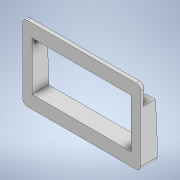
# Autodesk Inventor part: electricalCoverGasket02
Saved by Autodesk Inventor 2021.1 (Build 251245000, 245)
## iProperties
Created: 2020-08-29
Part Number: electricalCoverGasket02
Material: Generic
Document SubType Name: Modeling
Designer: robst
Density: 1 g/cm^3
Appearance: Default
Author: robst
Autodesk Inventor part; units mm, degrees
ref_plane "YZ Plane" through (0, 0, 0) normal (1, 0, 0) x (0, 1, 0)
ref_plane "XZ Plane" through (0, 0, 0) normal (0, 1, 0) x (-1, 0, 0)
sketch "Sketch1" plane through (0, 0, 0) normal (1, 0, 0) x (0, 1, 0)
  line L0 (0, 0) -> (0, 12.7)
  line L1 (0, 0) -> (-101.6, 0) construction
  arc A0 (-101.6, 0) -> (0, 0) centre (-50.8, 607.4796) ccw
  line L2 (-50.8, -2.1204) -> (-50.8, 0) construction
  line L3 (0, 12.7) -> (101.6, 12.7) construction
  arc A1 (0, 12.7) -> (101.6, 12.7) centre (50.8, 620.1796) ccw
  line L4 (19.685, 15.1842) -> (-57.785, 15.1842)
  line L5 (-57.785, 15.1842) -> (-57.785, -2.0803)
  line L6 (19.685, 15.1842) -> (19.685, 11.3742)
  dimension "d5" = 609.6
  dimension "d6" = 101.6
  dimension "d7" = 609.6
  dimension "d24" = 12.7
  dimension "d26" = 77.47
  dimension "d28" = 57.785
  dimension "d29" = 3.81
  constraints: 14 end point, 7 point on circle, 3 horizontal, 2 centre point, 2 perpendicular, 1 midpoint, 1 vertical
  measures "d5" radius of A0
  measures "d6" distance of L0.end L3.end
  measures "d7" radius of A1
  measures "d24" distance of L0.start L0.end
  measures "d26" distance of L4.start L4.end
  measures "d28" distance between parallel lines of L0 L5
  measures "d29" distance of L4.start L6.end
extrude "Extrusion3" add sketch "Sketch1" along normal mid plane 122.428
sketch "Sketch5" plane through (0, 0, 0) normal (0, 0, 1) x (1, 0, 0)
  line L0 (-61.214, 19.685) -> (61.214, 19.685) projected
  line L1 (-61.214, 0) -> (61.214, 0) projected
  line L2 (61.214, 0) -> (61.214, 19.685)
  line L3 (-61.214, 19.685) -> (-61.214, 0)
  line L4 (61.214, 12.065) -> (-61.214, 12.065) construction
  line L5 (-61.214, -57.785) -> (-61.214, 19.685) construction
  line L6 (21.5694, 8.255) -> (21.5694, 14.9734)
  line L7 (21.5694, 14.9734) -> (24.1259, 14.9734)
  line L8 (24.1259, 14.9734) -> (24.1259, 15.875)
  line L9 (24.1259, 15.875) -> (18.0002, 15.875)
  line L10 (18.0002, 15.875) -> (18.0002, 14.9734)
  line L11 (18.0002, 14.9734) -> (20.5567, 14.9734)
  line L12 (20.5567, 14.9734) -> (20.5567, 8.255)
  line L13 (20.5567, 8.255) -> (21.5694, 8.255)
  spline S0 degree 2 poles (11.8314, 15.0043) (11.3991, 14.498) (10.9175, 13.016) (10.9175, 12.065) knots 0 0 0 1 2 2 2
  spline S1 degree 2 poles (10.9175, 12.065) (10.9175, 11.1387) (11.3868, 9.6382) (11.8314, 9.1319) knots 0 0 0 1 2 2 2
  spline S2 degree 2 poles (11.8314, 9.1319) (12.3007, 8.6008) (13.5419, 8.0944) (14.289, 8.0944) knots 0 0 0 1 2 2 2
  spline S3 degree 2 poles (14.289, 8.0944) (15.0609, 8.0944) (16.2959, 8.6193) (16.7467, 9.1319) knots 0 0 0 1 2 2 2
  spline S4 degree 2 poles (16.7467, 9.1319) (17.1851, 9.6382) (17.6544, 11.1264) (17.6544, 12.065) knots 0 0 0 1 2 2 2
  spline S5 degree 2 poles (17.6544, 12.065) (17.6544, 13.0221) (17.179, 14.4794) (16.7405, 15.0043) knots 0 0 0 1 2 2 2
  spline S6 degree 2 poles (16.7405, 15.0043) (16.2959, 15.5107) (15.0547, 16.0356) (14.289, 16.0356) knots 0 0 0 1 2 2 2
  spline S7 degree 2 poles (14.289, 16.0356) (13.511, 16.0356) (12.2636, 15.4921) (11.8314, 15.0043) knots 0 0 0 1 2 2 2
  spline S8 degree 2 poles (11.9734, 12.065) (11.9734, 12.8184) (12.3007, 13.9854) (12.5971, 14.3683) knots 0 0 0 1 2 2 2
  spline S9 degree 2 poles (12.5971, 14.3683) (12.8997, 14.7635) (13.7518, 15.1587) (14.2829, 15.1587) knots 0 0 0 1 2 2 2
  spline S10 degree 2 poles (14.2829, 15.1587) (14.8324, 15.1587) (15.6599, 14.7758) (15.9748, 14.3683) knots 0 0 0 1 2 2 2
  spline S11 degree 2 poles (15.9748, 14.3683) (16.2774, 13.9793) (16.5985, 12.806) (16.5985, 12.065) knots 0 0 0 1 2 2 2
  spline S12 degree 2 poles (16.5985, 12.065) (16.5985, 10.5645) (15.3388, 8.9713) (14.2829, 8.9713) knots 0 0 0 1 2 2 2
  spline S13 degree 2 poles (14.2829, 8.9713) (13.2269, 8.9713) (11.9734, 10.5645) (11.9734, 12.065) knots 0 0 0 1 2 2 2
  spline S14 degree 2 poles (4.9894, 13.5779) (4.9894, 13.0839) (5.3414, 12.1947) (5.6563, 11.8859) knots 0 0 0 1 2 2 2
  spline S15 degree 2 poles (5.6563, 11.8859) (6.0515, 11.4969) (7.1198, 11.0955) (7.9349, 11.0955) knots 0 0 0 1 2 2 2
  line L14 (7.9349, 11.0955) -> (8.7933, 11.0955)
  line L15 (8.7933, 11.0955) -> (8.7933, 8.255)
  line L16 (8.7933, 8.255) -> (9.806, 8.255)
  line L17 (9.806, 8.255) -> (9.806, 15.875)
  line L18 (9.806, 15.875) -> (7.8917, 15.875)
  spline S16 degree 2 poles (7.8917, 15.875) (7.2124, 15.875) (6.2615, 15.6527) (5.8972, 15.3995) knots 0 0 0 1 2 2 2
  spline S17 degree 2 poles (5.8972, 15.3995) (5.4711, 15.1093) (4.9894, 14.2139) (4.9894, 13.5779) knots 0 0 0 1 2 2 2
  spline S18 degree 2 poles (6.0454, 13.547) (6.0454, 13.9422) (6.3171, 14.5227) (6.5949, 14.7079) knots 0 0 0 1 2 2 2
  spline S19 degree 2 poles (6.5949, 14.7079) (6.8358, 14.8685) (7.478, 14.9981) (7.9535, 14.9981) knots 0 0 0 1 2 2 2
  line L19 (7.9535, 14.9981) -> (8.7933, 14.9981)
  line L20 (8.7933, 14.9981) -> (8.7933, 11.96)
  line L21 (8.7933, 11.96) -> (8.1017, 11.96)
  spline S20 degree 2 poles (8.1017, 11.96) (7.4841, 11.96) (6.7246, 12.1576) (6.4776, 12.417) knots 0 0 0 1 2 2 2
  spline S21 degree 2 poles (6.4776, 12.417) (6.2491, 12.6455) (6.0454, 13.1827) (6.0454, 13.547) knots 0 0 0 1 2 2 2
  line L22 (1.0745, 16.2146) -> (4.057, 6.6001)
  line L23 (4.057, 6.6001) -> (4.9215, 6.6001)
  line L24 (4.9215, 6.6001) -> (1.9513, 16.2146)
  line L25 (1.9513, 16.2146) -> (1.0745, 16.2146)
  spline S22 degree 2 poles (-5.15, 10.5953) (-5.15, 10.0272) (-4.7177, 9.1566) (-4.3596, 8.8725) knots 0 0 0 1 2 2 2
  spline S23 degree 2 poles (-4.3596, 8.8725) (-3.9273, 8.5391) (-2.9455, 8.255) (-2.1674, 8.255) knots 0 0 0 1 2 2 2
  line L26 (-2.1674, 8.255) -> (0.0185, 8.255)
  line L27 (0.0185, 8.255) -> (0.0185, 15.875)
  line L28 (0.0185, 15.875) -> (-2.0007, 15.875)
  spline S24 degree 2 poles (-2.0007, 15.875) (-2.8158, 15.875) (-3.6309, 15.77) (-4.0014, 15.5662) knots 0 0 0 1 2 2 2
  spline S25 degree 2 poles (-4.0014, 15.5662) (-4.4152, 15.3501) (-4.7918, 14.64) (-4.7918, 14.1583) knots 0 0 0 1 2 2 2
  spline S26 degree 2 poles (-4.7918, 14.1583) (-4.7918, 13.6211) (-4.2237, 12.769) (-3.7235, 12.5281) knots 0 0 0 1 2 2 2
  line L29 (-3.7235, 12.5281) -> (-3.7235, 12.4911)
  spline S27 degree 2 poles (-3.7235, 12.4911) (-4.4028, 12.3058) (-5.15, 11.324) (-5.15, 10.5953) knots 0 0 0 1 2 2 2
  spline S28 degree 2 poles (-4.0941, 10.5521) (-4.0941, 10.9844) (-3.8471, 11.5401) (-3.4765, 11.7377) knots 0 0 0 1 2 2 2
  spline S29 degree 2 poles (-3.4765, 11.7377) (-3.2357, 11.8612) (-2.6676, 11.9353) (-2.1427, 11.9353) knots 0 0 0 1 2 2 2
  line L30 (-2.1427, 11.9353) -> (-0.9942, 11.9353)
  line L31 (-0.9942, 11.9353) -> (-0.9942, 9.1195)
  line L32 (-0.9942, 9.1195) -> (-1.8155, 9.1195)
  spline S30 degree 2 poles (-1.8155, 9.1195) (-2.4824, 9.1195) (-3.2481, 9.243) (-3.5445, 9.4406) knots 0 0 0 1 2 2 2
  spline S31 degree 2 poles (-3.5445, 9.4406) (-3.8285, 9.6444) (-4.0941, 10.1507) (-4.0941, 10.5521) knots 0 0 0 1 2 2 2
  spline S32 degree 2 poles (-3.7359, 14.0163) (-3.7359, 14.288) (-3.5506, 14.6956) (-3.3469, 14.8129) knots 0 0 0 1 2 2 2
  spline S33 degree 2 poles (-3.3469, 14.8129) (-3.0999, 14.9487) (-2.5009, 15.0105) (-1.9637, 15.0105) knots 0 0 0 1 2 2 2
  line L33 (-1.9637, 15.0105) -> (-0.9942, 15.0105)
  line L34 (-0.9942, 15.0105) -> (-0.9942, 12.7813)
  line L35 (-0.9942, 12.7813) -> (-2.1427, 12.7813)
  spline S34 degree 2 poles (-2.1427, 12.7813) (-2.6182, 12.7813) (-3.069, 12.8801) (-3.3098, 13.0345) knots 0 0 0 1 2 2 2
  spline S35 degree 2 poles (-3.3098, 13.0345) (-3.5445, 13.1827) (-3.7359, 13.6582) (-3.7359, 14.0163) knots 0 0 0 1 2 2 2
  line L36 (-5.3352, 8.255) -> (-7.9041, 15.875)
  line L37 (-7.9041, 15.875) -> (-9.1514, 15.875)
  line L38 (-9.1514, 15.875) -> (-11.7202, 8.255)
  line L39 (-11.7202, 8.255) -> (-10.6519, 8.255)
  line L40 (-10.6519, 8.255) -> (-9.9603, 10.3854)
  line L41 (-9.9603, 10.3854) -> (-7.0519, 10.3854)
  line L42 (-7.0519, 10.3854) -> (-6.3603, 8.255)
  line L43 (-6.3603, 8.255) -> (-5.3352, 8.255)
  line L44 (-9.6825, 11.2499) -> (-8.503, 14.8376)
  line L45 (-8.503, 14.8376) -> (-7.3298, 11.2499)
  line L46 (-7.3298, 11.2499) -> (-9.6825, 11.2499)
  spline S36 degree 2 poles (-15.5179, 8.1191) (-14.7769, 8.1191) (-13.5233, 8.6193) (-13.0664, 9.1195) knots 0 0 0 1 2 2 2
  spline S37 degree 2 poles (-13.0664, 9.1195) (-12.6094, 9.6135) (-12.1093, 11.0955) (-12.1093, 12.0588) knots 0 0 0 1 2 2 2
  spline S38 degree 2 poles (-12.1093, 12.0588) (-12.1093, 13.016) (-12.5971, 14.4362) (-13.0602, 14.9611) knots 0 0 0 1 2 2 2
  spline S39 degree 2 poles (-13.0602, 14.9611) (-13.5172, 15.4736) (-14.7645, 16.0109) (-15.5364, 16.0109) knots 0 0 0 1 2 2 2
  spline S40 degree 2 poles (-15.5364, 16.0109) (-15.9193, 16.0109) (-16.5923, 15.8997) (-16.8764, 15.8132) knots 0 0 0 1 2 2 2
  spline S41 degree 2 poles (-16.8764, 15.8132) (-17.1234, 15.733) (-17.6359, 15.5045) (-17.8891, 15.3686) knots 0 0 0 1 2 2 2
  line L47 (-17.8891, 15.3686) -> (-17.8891, 14.146)
  line L48 (-17.8891, 14.146) -> (-17.8088, 14.146)
  spline S42 degree 2 poles (-17.8088, 14.146) (-17.673, 14.2695) (-17.2531, 14.6153) (-16.9505, 14.782) knots 0 0 0 1 2 2 2
  spline S43 degree 2 poles (-16.9505, 14.782) (-16.6603, 14.9426) (-15.9748, 15.1463) (-15.5302, 15.1463) knots 0 0 0 1 2 2 2
  spline S44 degree 2 poles (-15.5302, 15.1463) (-15.0424, 15.1463) (-14.1717, 14.745) (-13.8444, 14.3621) knots 0 0 0 1 2 2 2
  spline S45 degree 2 poles (-13.8444, 14.3621) (-13.5233, 13.9731) (-13.1652, 12.7937) (-13.1652, 12.0588) knots 0 0 0 1 2 2 2
  spline S46 degree 2 poles (-13.1652, 12.0588) (-13.1652, 11.2746) (-13.5419, 10.1446) (-13.8691, 9.7555) knots 0 0 0 1 2 2 2
  spline S47 degree 2 poles (-13.8691, 9.7555) (-14.1902, 9.3789) (-15.0486, 8.996) (-15.5302, 8.996) knots 0 0 0 1 2 2 2
  spline S48 degree 2 poles (-15.5302, 8.996) (-15.9687, 8.996) (-16.7158, 9.2121) (-17.0061, 9.3727) knots 0 0 0 1 2 2 2
  spline S49 degree 2 poles (-17.0061, 9.3727) (-17.2839, 9.5332) (-17.6977, 9.8667) (-17.815, 9.984) knots 0 0 0 1 2 2 2
  line L49 (-17.815, 9.984) -> (-17.8891, 9.984)
  line L50 (-17.8891, 9.984) -> (-17.8891, 8.7737)
  spline S50 degree 2 poles (-17.8891, 8.7737) (-17.6359, 8.6564) (-17.1913, 8.4403) (-16.8764, 8.3415) knots 0 0 0 1 2 2 2
  spline S51 degree 2 poles (-16.8764, 8.3415) (-16.5429, 8.2303) (-15.9748, 8.1191) (-15.5179, 8.1191) knots 0 0 0 1 2 2 2
  line L51 (-24.3914, 8.255) -> (-23.0761, 8.255)
  line L52 (-23.0761, 8.255) -> (-20.2912, 11.7995)
  line L53 (-20.2912, 11.7995) -> (-19.8466, 11.2993)
  line L54 (-19.8466, 11.2993) -> (-19.8466, 8.255)
  line L55 (-19.8466, 8.255) -> (-18.8339, 8.255)
  line L56 (-18.8339, 8.255) -> (-18.8339, 15.875)
  line L57 (-18.8339, 15.875) -> (-19.8466, 15.875)
  line L58 (-19.8466, 15.875) -> (-19.8466, 12.3738)
  line L59 (-19.8466, 12.3738) -> (-22.9712, 15.875)
  line L60 (-22.9712, 15.875) -> (-24.2062, 15.875)
  line L61 (-24.2062, 15.875) -> (-21.0507, 12.4726)
  line L62 (-21.0507, 12.4726) -> (-24.3914, 8.255)
  point P0 (0, 0)
  dimension "d41" = 7.62
  constraints: 6 end point, 1 horizontal
  measures "d41" distance between parallel lines of L4 L0
emboss "Emboss3" sketch "Sketch5" operation cut depth 1.016 direction (0, 0, -1) wrap yes faces at (20.4047, 10.9309, 11.8848) contours L13 L12 L11 L10 L9 L8 L7 L6 | S7 S6 S5 S4 S3 S2 S1 S0 | S17 S16 L18 L17 L16 L15 L14 S15 S14 | L25 L24 L23 L22 | S27 L29 S26 S25 S24 L28 L27 L26 S23 S22 | L43 L42 L41 L40 L39 L38 L37 L36 | S51 S50 L50 L49 S49 S48 S47 S46 S45 S44 S43 S42 L48 L47 S41 S40 S39 S38 S37 S36 | L62 L61 L60 L59 L58 L57 L56 L55 L54 L53 L52 L51
ref_plane "Work Plane3" through (0, -50.8, -2.1204) normal (0, 0, 1) x (1, 0, 0)
sketch "Sketch8" plane through (-61.214, -57.785, 15.1842) normal (0, 0, 1) x (1, 0, 0)
  line L0 (122.428, 57.785) -> (0, 57.785) projected
  line L1 (61.214, 57.785) -> (61.214, 0) construction
  line L2 (0, 0) -> (122.428, 0) construction
  line L3 (9.779, 13.335) -> (112.649, 13.335)
  line L4 (112.649, 13.335) -> (112.649, 64.135)
  line L5 (112.649, 64.135) -> (9.779, 64.135)
  line L6 (9.779, 64.135) -> (9.779, 13.335)
  line L7 (9.779, 13.335) -> (112.649, 64.135) construction
  line L8 (112.649, 13.335) -> (9.779, 64.135) construction
  point P0 (61.214, 38.735)
  dimension "d36" = 50.8
  dimension "d37" = 102.87
  dimension "d38" = 13.335
  constraints: 14 end point, 3 midpoint, 2 parallel, 2 perpendicular, 1 point on line
  measures "d36" distance of L5.end L3.start
  measures "d37" distance between parallel lines of L4 L6
  measures "d38" distance between parallel lines of L2 L3
extrude "Extrusion4" cut sketch "Sketch8" against normal through all
sketch "Sketch9" plane through (0, -50.8, -2.1204) normal (0, 0, 1) x (1, 0, 0)
  line L0 (-61.214, -6.985) -> (61.214, -6.985) projected
  line L1 (-51.435, 6.35) -> (51.435, 6.35) projected
  line L2 (-51.435, 6.35) -> (-51.435, 57.15) construction
  line L3 (-51.435, 6.35) -> (-51.435, -6.985) construction
  line L4 (-61.214, -6.985) -> (61.214, -6.985) construction
  line L5 (51.435, 6.35) -> (-51.435, 6.35) construction
  line L6 (51.435, 6.35) -> (51.435, -6.985) construction
  line L7 (51.435, -0.3175) -> (-51.435, -0.3175) construction
  spline S0 degree 2 poles (7.604, -2.0321) (7.604, -2.6949) (8.1083, -3.7107) (8.5262, -4.0421) knots 0 0 0 1 2 2 2
  spline S1 degree 2 poles (8.5262, -4.0421) (9.0305, -4.4311) (10.176, -4.7625) (11.0837, -4.7625) knots 0 0 0 1 2 2 2
  line L8 (11.0837, -4.7625) -> (13.634, -4.7625)
  line L9 (13.634, -4.7625) -> (13.634, 4.1275)
  line L10 (13.634, 4.1275) -> (11.2782, 4.1275)
  spline S2 degree 2 poles (11.2782, 4.1275) (10.3272, 4.1275) (9.3763, 4.005) (8.944, 3.7673) knots 0 0 0 1 2 2 2
  spline S3 degree 2 poles (8.944, 3.7673) (8.4613, 3.5151) (8.0219, 2.6867) (8.0219, 2.1247) knots 0 0 0 1 2 2 2
  spline S4 degree 2 poles (8.0219, 2.1247) (8.0219, 1.498) (8.6847, 0.5038) (9.2682, 0.2228) knots 0 0 0 1 2 2 2
  line L11 (9.2682, 0.2228) -> (9.2682, 0.1796)
  spline S5 degree 2 poles (9.2682, 0.1796) (8.4758, -0.0365) (7.604, -1.182) (7.604, -2.0321) knots 0 0 0 1 2 2 2
  spline S6 degree 2 poles (8.836, -2.0825) (8.836, -1.5782) (9.1241, -0.9299) (9.5564, -0.6993) knots 0 0 0 1 2 2 2
  spline S7 degree 2 poles (9.5564, -0.6993) (9.8374, -0.5552) (10.5001, -0.4688) (11.1125, -0.4688) knots 0 0 0 1 2 2 2
  line L12 (11.1125, -0.4688) -> (12.4525, -0.4688)
  line L13 (12.4525, -0.4688) -> (12.4525, -3.7539)
  line L14 (12.4525, -3.7539) -> (11.4943, -3.7539)
  spline S8 degree 2 poles (11.4943, -3.7539) (10.7163, -3.7539) (9.8229, -3.6098) (9.4771, -3.3793) knots 0 0 0 1 2 2 2
  spline S9 degree 2 poles (9.4771, -3.3793) (9.1457, -3.1416) (8.836, -2.5508) (8.836, -2.0825) knots 0 0 0 1 2 2 2
  spline S10 degree 2 poles (9.2538, 1.959) (9.2538, 2.276) (9.4699, 2.7515) (9.7077, 2.8884) knots 0 0 0 1 2 2 2
  spline S11 degree 2 poles (9.7077, 2.8884) (9.9958, 3.0469) (10.6947, 3.1189) (11.3214, 3.1189) knots 0 0 0 1 2 2 2
  line L15 (11.3214, 3.1189) -> (12.4525, 3.1189)
  line L16 (12.4525, 3.1189) -> (12.4525, 0.5182)
  line L17 (12.4525, 0.5182) -> (11.1125, 0.5182)
  spline S12 degree 2 poles (11.1125, 0.5182) (10.5578, 0.5182) (10.0319, 0.6335) (9.7509, 0.8136) knots 0 0 0 1 2 2 2
  spline S13 degree 2 poles (9.7509, 0.8136) (9.4771, 0.9865) (9.2538, 1.5412) (9.2538, 1.959) knots 0 0 0 1 2 2 2
  line L18 (7.3879, -4.7625) -> (4.391, 4.1275)
  line L19 (4.391, 4.1275) -> (2.9357, 4.1275)
  line L20 (2.9357, 4.1275) -> (-0.0612, -4.7625)
  line L21 (-0.0612, -4.7625) -> (1.1851, -4.7625)
  line L22 (1.1851, -4.7625) -> (1.992, -2.277)
  line L23 (1.992, -2.277) -> (5.3851, -2.277)
  line L24 (5.3851, -2.277) -> (6.192, -4.7625)
  line L25 (6.192, -4.7625) -> (7.3879, -4.7625)
  line L26 (2.3162, -1.2685) -> (3.6922, 2.9172)
  line L27 (3.6922, 2.9172) -> (5.061, -1.2685)
  line L28 (5.061, -1.2685) -> (2.3162, -1.2685)
  spline S14 degree 2 poles (-4.4918, -4.921) (-3.6273, -4.921) (-2.1649, -4.3375) (-1.6318, -3.7539) knots 0 0 0 1 2 2 2
  spline S15 degree 2 poles (-1.6318, -3.7539) (-1.0986, -3.1776) (-0.5151, -1.4486) (-0.5151, -0.3247) knots 0 0 0 1 2 2 2
  spline S16 degree 2 poles (-0.5151, -0.3247) (-0.5151, 0.7919) (-1.0842, 2.4489) (-1.6246, 3.0613) knots 0 0 0 1 2 2 2
  spline S17 degree 2 poles (-1.6246, 3.0613) (-2.1577, 3.6592) (-3.6129, 4.286) (-4.5134, 4.286) knots 0 0 0 1 2 2 2
  spline S18 degree 2 poles (-4.5134, 4.286) (-4.9601, 4.286) (-5.7454, 4.1563) (-6.0768, 4.0555) knots 0 0 0 1 2 2 2
  spline S19 degree 2 poles (-6.0768, 4.0555) (-6.3649, 3.9618) (-6.9629, 3.6952) (-7.2582, 3.5368) knots 0 0 0 1 2 2 2
  line L29 (-7.2582, 3.5368) -> (-7.2582, 2.1103)
  line L30 (-7.2582, 2.1103) -> (-7.1646, 2.1103)
  spline S20 degree 2 poles (-7.1646, 2.1103) (-7.0061, 2.2544) (-6.5162, 2.6578) (-6.1632, 2.8524) knots 0 0 0 1 2 2 2
  spline S21 degree 2 poles (-6.1632, 2.8524) (-5.8246, 3.0397) (-5.0249, 3.2774) (-4.5062, 3.2774) knots 0 0 0 1 2 2 2
  spline S22 degree 2 poles (-4.5062, 3.2774) (-3.9371, 3.2774) (-2.9213, 2.8091) (-2.5395, 2.3625) knots 0 0 0 1 2 2 2
  spline S23 degree 2 poles (-2.5395, 2.3625) (-2.1649, 1.9086) (-1.747, 0.5326) (-1.747, -0.3247) knots 0 0 0 1 2 2 2
  spline S24 degree 2 poles (-1.747, -0.3247) (-1.747, -1.2396) (-2.1865, -2.558) (-2.5683, -3.0119) knots 0 0 0 1 2 2 2
  spline S25 degree 2 poles (-2.5683, -3.0119) (-2.9429, -3.4513) (-3.9443, -3.898) (-4.5062, -3.898) knots 0 0 0 1 2 2 2
  spline S26 degree 2 poles (-4.5062, -3.898) (-5.0177, -3.898) (-5.8894, -3.6458) (-6.228, -3.4585) knots 0 0 0 1 2 2 2
  spline S27 degree 2 poles (-6.228, -3.4585) (-6.5522, -3.2712) (-7.0349, -2.8822) (-7.1718, -2.7453) knots 0 0 0 1 2 2 2
  line L31 (-7.1718, -2.7453) -> (-7.2582, -2.7453)
  line L32 (-7.2582, -2.7453) -> (-7.2582, -4.1573)
  spline S28 degree 2 poles (-7.2582, -4.1573) (-6.9629, -4.2942) (-6.4442, -4.5464) (-6.0768, -4.6616) knots 0 0 0 1 2 2 2
  spline S29 degree 2 poles (-6.0768, -4.6616) (-5.6877, -4.7913) (-5.0249, -4.921) (-4.4918, -4.921) knots 0 0 0 1 2 2 2
  line L33 (-14.8443, -4.7625) -> (-13.3098, -4.7625)
  line L34 (-13.3098, -4.7625) -> (-10.0607, -0.6273)
  line L35 (-10.0607, -0.6273) -> (-9.542, -1.2108)
  line L36 (-9.542, -1.2108) -> (-9.542, -4.7625)
  line L37 (-9.542, -4.7625) -> (-8.3605, -4.7625)
  line L38 (-8.3605, -4.7625) -> (-8.3605, 4.1275)
  line L39 (-8.3605, 4.1275) -> (-9.542, 4.1275)
  line L40 (-9.542, 4.1275) -> (-9.542, 0.0427)
  line L41 (-9.542, 0.0427) -> (-13.1873, 4.1275)
  line L42 (-13.1873, 4.1275) -> (-14.6282, 4.1275)
  line L43 (-14.6282, 4.1275) -> (-10.9468, 0.158)
  line L44 (-10.9468, 0.158) -> (-14.8443, -4.7625)
  point P0 (0, 50.8)
  constraints: 6 end point, 2 midpoint, 2 perpendicular, 2 point on line, 1 horizontal
emboss "Emboss5" sketch "Sketch9" operation cut depth 1.016 direction (0, 0, -1) wrap yes faces at (17.145, -53.3401, -2.1151)
fillet "Fillet1" radius 4.7625 4 edges at (-61.214, 19.685, 13.2792) (-61.214, -57.785, 6.552) (61.214, -57.785, 6.552) (61.214, 19.685, 13.2792)
equation "\"d5\" = radiusOfCurvature"
equation "\"d6\" = sidingHeight"
equation "\"d7\" = radiusOfCurvature"
equation "\"d24\" = sidingDepth"
equation "\"d26\" = coverHeight"
equation "\"d29\" = partMinDepth"
equation "\"d30\" = coverWidth"
equation "\"d32\" = textDepth"
equation "\"d42\" = textDepth"
equation "\"d44\" = filletRadiusAroundEdges"
equation "\"sidingHeight\" = 101.6"
equation "\"sidingDepth\" = 12.7"
equation "\"radiusOfCurvature\" = 609.6"
equation "\"partMinDepth\" = 3.81"
equation "\"coverHeight\" = 77.47"
equation "\"coverWidth\" = 122.428"
equation "\"electricalPlugHeight\" = 38.1"
equation "\"insideHoleWidth\" = 102.87"
equation "\"insideHoleHeight\" = 50.8"
equation "\"textDepth\" = 1.016"
equation "\"textCenterLine\" = 6.6675"
equation "\"filletRadiusAroundEdges\" = 4.7625"
body "Solid1"
body "Solid2"
